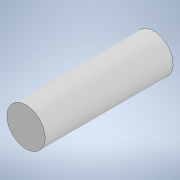
# Autodesk Inventor part: CilindroHidraulico_1
Saved by Autodesk Inventor 2021 (Build 250183000, 183)
## iProperties
Created: 2021-07-12
Part Number: CilindroHidraulico_1
Material: Generic
Document SubType Name: Modeling
Designer: Nelson
Density: 1 g/cm^3
Appearance: Default
Author: Nelson
Autodesk Inventor part; units mm, degrees
ref_plane "YZ Plane" through (0, 0, 0) normal (1, 0, 0) x (0, 1, 0)
ref_plane "XZ Plane" through (0, 0, 0) normal (0, 1, 0) x (-1, 0, 0)
ref_plane "XY Plane" through (0, 0, 0) normal (0, 0, 1) x (1, 0, 0)
sketch "Sketch2" plane through (0, 0, 0) normal (1, 0, 0) x (0, 1, 0)
  line L0 (0, 0) -> (50, 0)
  line L1 (50, -335) -> (0, -335)
  line L2 (0, -335) -> (0, 0)
  line L3 (0, 0) -> (50, 0)
  line L4 (50, 0) -> (50, -26)
  line L5 (50, -26) -> (12.5, -26)
  line L6 (50, -335) -> (50, -248)
  line L7 (50, -248) -> (12.5, -248)
  line L8 (12.5, -26) -> (12.5, -248)
  line L9 (0, -335) -> (0, -465) construction
  dimension "d4" = 50
  dimension "d7" = 335
  dimension "d8" = 50
  dimension "d9" = 26
  dimension "d10" = 37.5
  dimension "d12" = 37.5
  dimension "d20" = 87
  constraints: 20 end point, 2 horizontal, 2 parallel, 2 perpendicular, 2 vertical, 1 collinear
  measures "d4" distance of L1.start L1.end
  measures "d7" distance of L1.end L0.start
  measures "d8" distance of L0.start L0.end
  measures "d9" distance of L0.end L4.end
  measures "d10" distance of L4.end L5.end
  measures "d12" distance of L6.end L7.end
  measures "d20" distance of L1.start L6.end
revolve "Revolution1" add sketch "Sketch2" angle 360 about axis through (0, 50, 0) along (0, 0, -1)
sketch "Sketch3" plane through (0, 50, -335) normal (0, 0, -1) x (-1, 0, 0)
  circle A0 centre (0, 0) radius 28
  point P0 (0, -50)
  dimension "d14" = 56
  constraints: 1 centre point
  measures "d14" diameter of A0
extrude "Extrusion2" cut sketch "Sketch3" against normal blind 309
equation "\"d4\" = d8"
equation "\"d12\" = d10"
body "Solid2"
